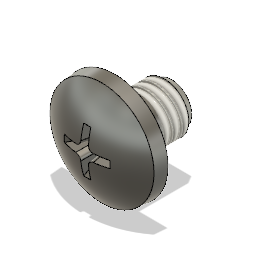
in12_Nixie_Clock_Case v41 (Autodesk Fusion 360 archive; units mm, degrees)
design "Type I Cross Recessed Binding Head Machine Screw ANSI B18.6.3 4-48 UNF x 0.125 Steel Grade 2 Plain"
description: Type I Cross Recessed Binding Head Machine Screw ANSI B18.6.3 4-48 UNF x 0.125
Autodesk Fusion 360 part; units mm, degrees
sketch "Sketch1" plane through (0, 0, 0) normal (0, 1, 0) x (1, 0, 0)
  line L0 (-1.4224, 0) -> (-1.4224, 3.175)
  line L1 (-1.4224, 3.175) -> (0, 3.175)
  line L2 (0, 3.175) -> (0, -1.7272)
  line L3 (-1.4224, 0) -> (-2.9845, 0)
  line L4 (-2.9845, 0) -> (-2.9206, -0.7299)
  arc A0 (-2.9206, -0.7299) -> (0, -1.7272) centre (0, 3.048) ccw
  dimension "d9" = 2.8448
  dimension "d66" = 5.969
  dimension "d67" = 1.7272
  dimension "d68" = 3.175
  dimension "d70" = 4.7752
  dimension "d86" = 85
  constraint perpendicular L0 L1
  constraint collinear origin L2.end L1.end
  constraint perpendicular L0 L3
  constraint coincident origin L3
  constraint vertical L0
  constraint vertical L2
  constraint coincident L2 A0.centre
  measures "d67" vertical distance of L2.end L3.end
  measures "d68" distance of origin L1.end
  measures "d70" radius of A0
  measures "d86" angle of L3 L4
revolve "Revolve1" add sketch "Sketch1" angle 360 about axis through (0, 0, -3.175) along (0, 0, 1)
ref_plane "WorkPlane1" through (0, 0, 1.7272) normal (0, 0, 1) x (1, 0, 0)
sketch "Sketch2" plane through (0, 0, 1.7272) normal (0, 0, 1) x (1, 0, 0)
  circle A0 centre (0, 0) radius 3
  line L0 (-0.2159, 1.4097) -> (-0.2159, 0.2159)
  line L1 (-0.2159, 0.2159) -> (-1.4097, 0.2159)
  line L2 (0, 0) -> (0, 1.4097) construction
  line L3 (0.2159, 0.2159) -> (1.4097, 0.2159)
  line L4 (0.2159, 1.4097) -> (0.2159, 0.2159)
  line L5 (0.2159, -0.2159) -> (1.4097, -0.2159)
  line L6 (0.2159, -1.4097) -> (0.2159, -0.2159)
  line L7 (-0.2159, -1.4097) -> (-0.2159, -0.2159)
  line L8 (-0.2159, -0.2159) -> (-1.4097, -0.2159)
  line L9 (-0.2159, 1.4097) -> (0.2159, 1.4097)
  line L10 (-1.4097, 0.2159) -> (-1.4097, -0.2159)
  line L11 (-0.2159, -1.4097) -> (0.2159, -1.4097)
  line L12 (1.4097, -0.2159) -> (1.4097, 0.2159)
  line L13 (1.75, 0) -> (22.5, 0)
  circle A1 centre (0, 0) radius 1.5
  dimension "d22" = 0.4318
  dimension "d57" = 2.8194
  constraint perpendicular L0 L1
  constraint coincident A0.centre L2.start
  constraint symmetric L0.start L2 L4.start
  constraint symmetric L0.end L2 L3.start
  constraint symmetric L1.end L2 L3.end
  constraint perpendicular L4 L9
  constraint perpendicular L8 L10
  constraint equal L9 L10
  constraint equal L0 L1
  constraint symmetric L1 L8 L13
  constraint horizontal L0.start L2.end
  constraint vertical L2
  constraint symmetric L3 L5 L13
  constraint symmetric L2 L6 L7
  constraint symmetric L9 L11 L13
  constraint collinear L4 L6
  measures "d22" horizontal distance of L0.start L4.start
  measures "d57" distance of L10 L12
extrude "Extrude1" cut sketch "Sketch2" against normal blind 1.7272 draft -6 contours L0 L1 L3 L4 L5 L6 L7 L8 L9 L10 L11 L12
fillet "Fillet3" radius 0.2819 4 edges at (-0.1246, 0.1246, 0.8588) (0.1246, 0.1246, 0.8588) (0.1246, -0.1246, 0.8588) (-0.1246, -0.1246, 0.8588)
draft "Draft1" angle 30 neutral plane through (0, 0, 1.7272) pull (0, 0, 1) 4 faces at (1.3347, -0.0115, 1.0137) (-0.0115, 1.3347, 1.0137) (-1.2815, 0, 0.507) (-0.0115, -1.3347, 1.0137)
thread "Thread2" "ANSI Unified Screw Threads 0.112(#4) 4-48 UNF 2A" major diameter 2.7711 minor diameter 2.1946 pitch 0.5292 angle 60 resizes the face on face at (-1.4153, 0.1416, -1.0583) from (0, 0, -1.3228) to (0, 0, -3.175)
sketch "Sketch5" plane through (0, 0, 0) normal (0, 1, 0) x (1, 0, 0)
  line L0 (0, -1.75) -> (0, -22.5)
  line L1 (0, 3.175) -> (0, -1.7272)
  line L2 (0, 3.175) -> (-1.4508, 3.175)
  line L3 (-1.4508, 3.175) -> (-1.4508, 2.6458)
  line L4 (-1.4508, 2.6458) -> (-1.1354, 3.175)
  dimension "d98" = 1.1354
  dimension "d99" = 1.4508
  dimension "d100" = 0.5292
  constraint coincident L1.start L2.start
  constraint perpendicular L1 L2
  constraint perpendicular L2 L3
  constraint coincident L2 L4.end
  measures "d98" horizontal distance of origin L4.end
  measures "d99" horizontal distance of origin L2.end
  measures "d100" distance of L2.end L3.end
revolve "Revolve2" cut sketch "Sketch5" angle 360 about axis through (0, 0, -3.175) along (0, 0, 1)
equation "d9 = adsk_nomdia"
equation "d22 = adsk_slotw"
equation "d31 = -adsk_slotdepth"
equation "d57 = adsk_slotdia"
equation "d59 = adsk_slotdia * 0.1"
equation "d66 = adsk_headdia"
equation "d67 = adsk_headh"
equation "d68 = adsk_nomlen"
equation "d70 = adsk_headdia * 0.8"
equation "d71 = adsk_headh"
equation "adsk_nomlen = 0.125 in"
equation "adsk_headh = 0.068 in"
equation "adsk_headdia = 0.235 in"
equation "adsk_nomdia = 0.112 in"
equation "adsk_slotdia = 0.111 in"
equation "adsk_slotw = 0.017 in"
equation "adsk_slotdepth = 0.068 in"
equation "adsk_thrlen = 0.07292 in"
equation "adsk_startlen = 0.020833 in"
equation "adsk_endpointdia = 0.0894 in"
equation "d98 = adsk_endpointdia / 2"
equation "d99 = adsk_nomdia * 0.51"
equation "d100 = adsk_startlen"
